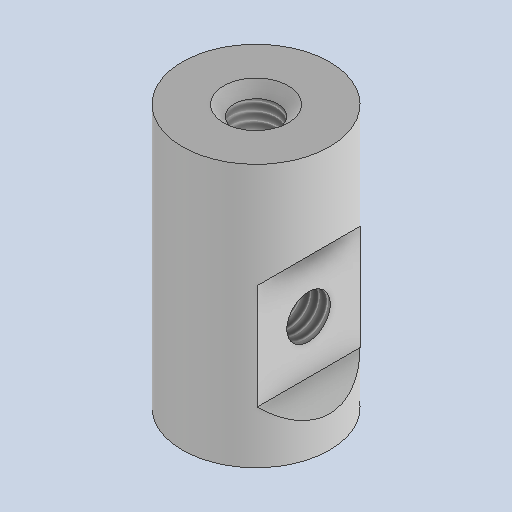
# Autodesk Inventor part: TS_V1_Fallmagazin_Schieberanbindung_int
Saved by Autodesk Inventor 2025.2 (Build 292293000, 293)
## iProperties
Created: 2025-06-13
Part Number: TS_V1_Fallmagazin_Schieberanbindung_int
Material: Generisch
Document SubType Name: Modeling
Designer: tino
Density: 1 g/cm^3
Appearance: Vorgabe
Author: tino
Autodesk Inventor part; units mm, degrees
ref_plane "XY Plane" through (0, 0, 0) normal (0, 0, 1) x (1, 0, 0)
sketch "Skizze1" plane through (0, 0, 0) normal (0, 0, 1) x (1, 0, 0)
  circle A0 centre (0, 0) radius 7
  dimension "d0" = 14
  constraints: 1 centre point, 1 coincident
  measures "d0" diameter of A0
extrude "Extrusion1" add sketch "Skizze1" along normal blind 25
sketch "Skizze2" plane through (0, 0, 25) normal (0, 0, 1) x (1, 0, 0)
  circle A0 centre (0, 0) radius 7 projected
hole "Bohrung1" at (0, 0, 25) direction (0, 0, -1) diameter 4.134 depth 11.5 tip angle 118 thread size "M5x0.8" class "6H" standard "ISO Metric profile"
chamfer "Fasen1" distance 1 angle 45 1 edges at (0, 2.067, 25)
ref_plane "Arbeitsebene1" through (-7, 0, 0) normal (1, 0, 0) x (0, 1, 0)
ref_plane "Arbeitsebene2" through (0, -7, 0) normal (0, 1, 0) x (-1, 0, 0)
ref_plane "Arbeitsebene3" through (7, 0, 0) normal (1, 0, 0) x (0, 1, 0)
sketch "Skizze6" plane through (7, 0, 0) normal (1, 0, 0) x (0, 1, 0)
  line L0 (-7, 0) -> (-7, 25) projected
  line L1 (7, 0) -> (7, 25) projected
  line L2 (-7, 5) -> (7, 5)
  line L3 (7, 5) -> (7, 15)
  line L4 (7, 15) -> (-7, 15)
  line L5 (-7, 15) -> (-7, 5)
  line L6 (7, 25) -> (-7, 25) projected
  point P0 (0, 0)
  point P1 (-7, 15)
  point P2 (7, 5)
  dimension "d29" = 10
  dimension "d30" = 10
  constraints: 8 end point, 2 parallel, 2 point on line, 1 horizontal, 1 perpendicular
  measures "d29" distance of L3.end L2.end
  measures "d30" distance between parallel lines of L6 L4
extrude "Extrusion4" cut sketch "Skizze6" against normal blind 2 contours L0 L4 L1 L2
sketch "Skizze7" plane through (5, 0, 0) normal (1, 0, 0) x (0, 0, -1)
  line L0 (-5, -4.899) -> (-5, 4.899) projected
  line L1 (0, 7) -> (0, -7) projected
  point P0 (0, 0)
  point P1 (-10, 0)
  point P2 (0, 0)
  point P3 (0, 0)
  point P4 (0, 0)
  dimension "d33" = 5
  constraints: 1 horizontal alignment, 1 midpoint
  measures "d33" distance from line of point (-10, 0) L0
hole "Bohrung3" at (5, 0, 10) direction (-1, 0, 0) diameter 4.134 end through all thread size "M5x0.8" class "6H" standard "ISO Metric profile"
ref_plane "Arbeitsebene4" through (0, 7, 0) normal (0, 1, 0) x (-1, 0, 0)
sketch "Skizze8" plane through (0, 7, 0) normal (0, 1, 0) x (-1, 0, 0)
  line L0 (-5, 5) -> (-5, 5) projected
  line L1 (-5, 7.933) -> (-5, 12.067) projected
  line L2 (-5, 5) -> (-5, 15) projected
  line L3 (-5, 15) -> (-5, 5) projected
  line L4 (-5, 15) -> (-7, 15) projected
  line L5 (-5, 15) -> (-5, 5) projected
  line L6 (-5, 5) -> (-5, 15) projected
  line L7 (-5, 15) -> (-5, 15) projected
  line L8 (-7, 5) -> (-5, 5) projected
  line L9 (-5, 5) -> (-7, 3)
  line L10 (-7, 0) -> (-7, 25) projected
  line L11 (-5, 5) -> (-2.1716, 5) construction
  line L12 (-7, 3) -> (-7, 5)
  line L13 (-5, 15) -> (-7, 17)
  line L14 (-5, 15) -> (-2.1716, 15) construction
  line L15 (-7, 17) -> (-7, 15)
  point P0 (0, 0)
  point P1 (-5, 24.433)
  point P2 (-5, 28.567)
  dimension "d42" = 135
  dimension "d43" = 135
  constraints: 12 end point, 2 equal length, 2 horizontal, 2 point on line, 1 collinear, 1 perpendicular
  measures "d42" angle of L9 L11
  measures "d43" angle of L14 L13
extrude "Extrusion5" cut sketch "Skizze8" against normal through all contours L9 L10 L8 | L4 L10 L13
